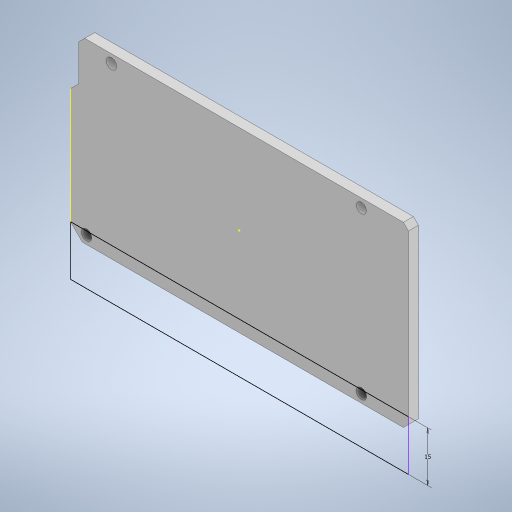
# Autodesk Inventor part: arduino_holder
Saved by Autodesk Inventor 2024 (Build 280153000, 153)
## iProperties
Created: 2026-01-02
Part Number: arduino_holder
Material: Generic
Document SubType Name: Modeling
Designer: schar
Density: 1 g/cm^3
Appearance: Default
Author: schar
Autodesk Inventor part; units mm, degrees
ref_plane "YZ Plane" through (0, 0, 0) normal (1, 0, 0) x (0, 1, 0)
ref_plane "XZ Plane" through (0, 0, 0) normal (0, 1, 0) x (-1, 0, 0)
ref_plane "Work Plane1" through (-47.244, -26.7081, 1.651) normal (0, 0, 1) x (1, 0, 0)
sketch "Sketch1" plane through (-47.244, -26.7081, 1.651) normal (0, 0, 1) x (1, 0, 0)
  line L0 (-3.556, 38.1762) -> (-3.556, 3.556) projected
  line L1 (-1.016, 40.7162) -> (-3.556, 38.1762) projected
  line L2 (-3.556, 38.1762) -> (-1.016, 40.7162)
  line L3 (0.7474, 53.4162) -> (-1.016, 51.6528) projected
  line L4 (-1.016, 40.7162) -> (-1.016, 51.6528)
  line L5 (-1.016, 51.6528) -> (0.7474, 53.4162)
  line L6 (98.044, 51.8922) -> (96.52, 53.4162) projected
  line L7 (0.7474, 53.4162) -> (96.52, 53.4162)
  line L8 (96.52, 53.4162) -> (98.044, 51.8922)
  line L9 (96.52, 0) -> (98.044, 1.524) projected
  line L10 (98.044, 51.8922) -> (98.044, 1.524)
  line L11 (98.044, 1.524) -> (96.52, 0)
  line L12 (0, 0) -> (-3.556, 3.556) projected
  line L13 (96.52, 0) -> (0, 0)
  line L14 (0, 0) -> (-3.556, 3.556)
  line L15 (-3.556, 3.556) -> (-3.556, 38.1762)
  circle A0 centre (8.7884, 50.8762) radius 1.5621 projected
  circle A1 centre (8.7884, 50.8762) radius 1.5
  circle A2 centre (83.9216, 50.8762) radius 1.5
  circle A3 centre (83.9216, 2.54) radius 1.5621 projected
  circle A4 centre (83.9216, 2.54) radius 1.5
  circle A5 centre (1.2954, 2.54) radius 1.5621 projected
  circle A6 centre (1.2954, 2.54) radius 1.5
  point P0 (47.244, 26.7081)
  dimension "d1" = 3
  dimension "d2" = 3
  dimension "d3" = 3
  dimension "d4" = 3
  constraints: 20 end point, 5 collinear, 4 centre point, 4 coincident, 3 perpendicular, 1 parallel, 1 vertical
  measures "d1" diameter of A1
  measures "d2" diameter of A2
  measures "d3" diameter of A4
  measures "d4" diameter of A6
extrude "Extrusion1" add sketch "Sketch1" along normal blind 3 contours L1 L4 L3 L7 L6 L10 L9 L13 L12 L0
sketch "Sketch2" plane through (-47.244, -26.7081, 4.651) normal (0, 0, 1) x (1, 0, 0)
  line L0 (-3.556, 38.1762) -> (-3.556, 3.556) projected
  line L1 (-3.556, 3.556) -> (98.044, 3.556)
  line L2 (98.044, 3.556) -> (98.044, -11.444)
  line L3 (98.044, -11.444) -> (-3.556, -11.444)
  line L4 (-3.556, -11.444) -> (-3.556, 3.556)
  point P0 (47.244, 26.7081)
  dimension "d7" = 15
  constraints: 8 end point, 2 parallel, 1 horizontal, 1 perpendicular
  measures "d7" distance of L1.end L2.end
body "Solid1"
